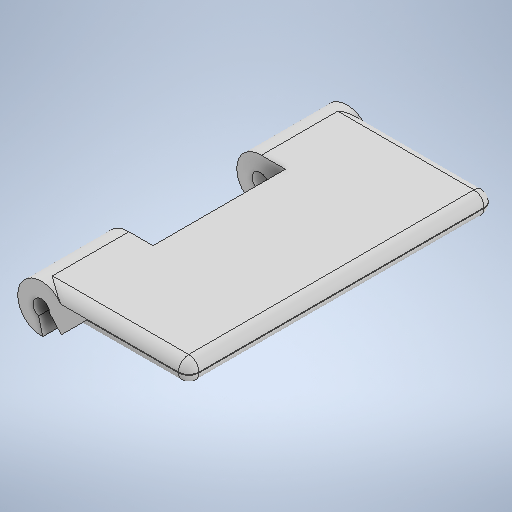
# Autodesk Inventor part: Pieza6
Saved by Autodesk Inventor 2025.1 (Build 291241020, 241B)
## iProperties
Created: 2024-11-25
Part Number: Pieza6
Material: Genérico
Document SubType Name: Modeling
Designer: ctamashiro
Density: 1 g/cm^3
Appearance: Valor por defecto
Author: ctamashiro
Autodesk Inventor part; units mm, degrees
ref_plane "YZ Plane" through (0, 0, 0) normal (1, 0, 0) x (0, 1, 0)
ref_plane "XZ Plane" through (0, 0, 0) normal (0, 1, 0) x (-1, 0, 0)
ref_plane "XY Plane" through (0, 0, 0) normal (0, 0, 1) x (1, 0, 0)
sketch "Boceto1" plane through (0, 0, 0) normal (0, 1, 0) x (-1, 0, 0)
  line L0 (-12.5, -30) -> (12.5, -30)
  line L1 (12.5, -30) -> (12.5, 30)
  line L2 (12.5, 30) -> (-12.5, 30)
  line L3 (-12.5, 30) -> (-12.5, -30)
  line L4 (-12.5, -30) -> (12.5, 30) construction
  line L5 (12.5, -30) -> (-12.5, 30) construction
  line L6 (61.5, -13) -> (11.5, -13)
  line L7 (11.5, -13) -> (11.5, 13)
  line L8 (11.5, 13) -> (61.5, 13)
  line L9 (61.5, 13) -> (61.5, -13)
  line L10 (12.5, 0) -> (11.5, 0) construction
  point P0 (0, 0)
  point P1 (12.5, 13)
  point P2 (12.5, -13)
  dimension "d0" = 25
  dimension "d1" = 60
  dimension "d8" = 50
  dimension "d9" = 26
  dimension "d10" = 1
  constraints: 22 end point, 4 midpoint, 4 parallel, 3 horizontal, 2 perpendicular
  measures "d0" distance of L2.end L1.end
  measures "d1" distance of L1.end L0.end
  measures "d8" distance of L7.end L8.end
  measures "d9" distance of L6.end L7.end
  measures "d10" distance of L10.end L10.start
extrude "Extrusión1" add sketch "Boceto1" along normal blind 5 contours L3 L2 L1 L8 L7 L6 L0 | L6 L7 L8 L1
sketch "Boceto2" plane through (-12.5, 0, 30) normal (0, 0, 1) x (1, 0, 0)
  circle A0 centre (-3.9208, 2.5) radius 1.65
  line L0 (0, 0) -> (0, 5) construction
  line L1 (0, 2.5) -> (-8.4797, 2.5) construction
  circle A1 centre (-3.9208, 2.5) radius 4.65
  line L2 (-2.2708, 2.5) -> (0, 0)
  line L3 (-2.2708, 2.5) -> (-26.7468, 29.4468) construction
  line L4 (-6.0334, 6.6424) -> (-3.6387, -2.1414)
  line L5 (0, 5) -> (25, 5) projected
  line L6 (-3.7417, 7.1465) -> (25, 7.1465)
  line L7 (25, 7.1465) -> (25, 5)
  line L8 (25, 5) -> (-3.7417, 5)
  line L9 (-3.7417, 5) -> (-3.7417, 7.1465)
  arc A2 (0, 0) -> (0.7292, 2.5) centre (-3.9208, 2.5) ccw
  line L10 (-6.0334, 6.6424) -> (-1.5623, -1.5075) construction
  point P0 (12.5, 0)
  point P1 (-4.481, 0.948)
  dimension "d4" = 3.3
  dimension "d5" = 3
  constraints: 18 end point, 10 point on circle, 5 point on line, 3 centre point, 2 coincident, 2 horizontal, 2 parallel, 1 collinear, 1 midpoint, 1 perpendicular
  measures "d4" diameter of A0
  measures "d5" radial gap between concentric circles of A0 A1
extrude "Extrusión2" add sketch "Boceto2" against normal blind 60 contours A0 L4 A1 L9 L8 L2 | A0 L4 A1 | L6 L7 L5 A1 | A1 L8 L9
extrude "Extrusión3" cut sketch "Boceto1" along normal through all both and the other way through all contours L6 L7 L8 L1 | L1 L8 L9 L6
sketch "Boceto3" plane through (-16.2417, 7.1465, 30) normal (0, 0, 1) x (1, 0, 0)
  line L0 (3.7417, -7.1465) -> (28.7417, -7.1465) projected
  line L1 (28.7417, -7.1465) -> (28.7417, 0) projected
  line L2 (3.7417, -7.1465) -> (28.7417, -7.1465)
  line L3 (28.7417, -7.1465) -> (28.7417, -4.1465)
  line L4 (28.7417, -4.1465) -> (3.7417, -4.1465)
  line L5 (3.7417, -4.1465) -> (3.7417, -7.1465)
  line L6 (3.7417, -7.1465) -> (6.7417, -4.1465)
  line L7 (3.7417, -7.1465) -> (7.9843, -7.1465) construction
  point P0 (16.2417, -7.1465)
  dimension "d13" = 3
  dimension "d16" = 45
  constraints: 12 end point, 2 horizontal, 2 parallel, 2 point on line, 1 equal length, 1 perpendicular
  measures "d13" distance of L3.end L2.end
  measures "d16" angle of L7 L6
extrude "Extrusión4" cut sketch "Boceto3" against normal blind 60 contours L6 L4 L1 L0
extrude "Extrusión5" cut sketch "Boceto3" along normal up to surface (26 mm away) from surface at -43 contours L5 L4 L6
fillet "Empalme1" radius 2 2 edges at (12.5, 7.1465, 0) (12.5, 3, 0)
fillet "Empalme2" radius 2 10 edges at (11.9142, 6.5608, 30) (12.5, 5.0733, 30) (11.9142, 3.5858, 30) (0.5, 3, 30) (-2.8708, 7.1465, 30) (11.9142, 6.5608, -30) (12.5, 5.0733, -30) (11.9142, 3.5858, -30) (0.5, 3, -30) (-2.8708, 7.1465, -30)
